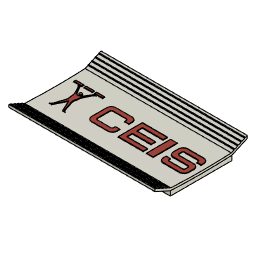
Pen_holder_ceis (Autodesk Fusion 360 design; units mm, degrees)
Autodesk Fusion 360 part; units mm, degrees
sketch "Schizzo3" plane through (0, 0, 0) normal (0, 0, 1) x (1, 0, 0)
  line L0 (0, 0) -> (190, 0)
  line L1 (190, 0) -> (190, 80)
  line L2 (190, 80) -> (0, 80)
  line L3 (0, 80) -> (0, 0)
  dimension "d7" = 80
  dimension "d8" = 190
  constraint horizontal L0
  constraint vertical L1
  constraint horizontal L2
  constraint vertical L3
  constraint coincident L0.start L3.end
  measures "d7" distance of L0.start L2.end
  measures "d8" distance of L1.end L2.end
extrude "Estrusione2" add sketch "Schizzo3" along normal blind 6 makes body 1
sketch "Schizzo4" plane through (190, 0, 0) normal (1, 0, 0) x (0, 1, 0)
  line L0 (0, 0) -> (80, 0)
  line L1 (80, 0) -> (80, 6)
  line L2 (80, 6) -> (0, 6)
  line L3 (0, 6) -> (0, 0)
  line L4 (0, 6) -> (0, 5)
  line L5 (40, 5) -> (40, 9)
  line L6 (-6.5555, 6.3549) -> (30, 25)
  line L7 (30, 25) -> (86.5555, 6.3549)
  arc A0 (-6.5555, 6.3549) -> (86.5555, 6.3549) centre (40, 805.5001) ccw
  constraint coincident L2.end L3.start
  constraint coincident L3 L4.end
  constraint perpendicular L2 L4
  constraint perpendicular L2 L5
  constraint coincident L5.start A0
  constraint coincident L1.end A0
  constraint coincident L2.end A0
extrude "Estrusione3" cut sketch "Schizzo4" against normal through all contours L2 L5 A0 | L2 L6 L7 A0 | L2 L5 A0 bodies 1
sketch "Schizzo5" plane through (190, 0, 0) normal (1, 0, 0) x (0, 1, 0)
  line L0 (80, 0) -> (80, 6)
  line L1 (0, 0) -> (-20, 0)
  line L2 (-20, 0) -> (-20, 15)
  line L3 (80, 0) -> (100, 0)
  line L4 (100, 0) -> (100, 15)
  line L5 (-20, 15) -> (0, 6)
  line L6 (100, 15) -> (80, 6)
  spline S0 degree 5 poles (0, 6) (1.6, 5.9242) (4.8, 5.7791) (9.6, 5.5813) (16, 5.3581) (24, 5.1509) (32, 5.0221) (40, 4.978) (48, 5.0221) (56, 5.1509) (64, 5.3581) (70.4, 5.5813) (75.2, 5.7791) (78.4, 5.9242) (80, 6) knots 0 0 0 0 0 0 0.1 0.2 0.3 0.4 0.5 0.6 0.7 0.8 0.9 1 1 1 1 1 1
  line L7 (-20, 15) -> (-20, 18.2898)
  line L8 (100, 15) -> (100, 18.2898)
  line L9 (-18.7689, 17.7358) -> (0.7109, 8.9698)
  spline S1 degree 3 poles (0.7109, 8.9698) (18.3427, 8.1444) (35.9568, 7.8068) (53.5771, 8.1239) (62.1442, 8.2781) (70.7163, 8.5685) (79.2891, 8.9698) knots 0.007133 0.007133 0.007133 0.007133 0.670389 0.670389 0.670389 0.992867 0.992867 0.992867 0.992867
  line L10 (98.7689, 17.7358) -> (79.2891, 8.9698)
  line L11 (98.7689, 17.7358) -> (100, 18.2898)
  line L12 (-18.7689, 17.7358) -> (-20, 18.2898)
  line L13 (0.7109, 8.9698) -> (-2.9367, 10.6113)
  line L14 (-2.9367, 10.6113) -> (-2.7316, 11.0673)
  line L15 (-2.7316, 11.0673) -> (-3.6435, 11.4776)
  line L16 (-3.6435, 11.4776) -> (-3.8487, 11.0217)
  line L17 (-3.8487, 11.0217) -> (-7.4964, 12.6631)
  line L18 (-7.4964, 12.6631) -> (-7.2912, 13.1191)
  line L19 (-7.2912, 13.1191) -> (-8.2031, 13.5294)
  line L20 (-8.2031, 13.5294) -> (-8.4083, 13.0735)
  line L21 (-8.4083, 13.0735) -> (-12.056, 14.7149)
  line L22 (-12.056, 14.7149) -> (-11.8508, 15.1709)
  line L23 (-11.8508, 15.1709) -> (-12.7627, 15.5813)
  line L24 (-12.7627, 15.5813) -> (-12.9679, 15.1253)
  line L25 (-12.9679, 15.1253) -> (-16.6156, 16.7668)
  line L26 (-16.6156, 16.7668) -> (-16.4104, 17.2227)
  line L27 (-16.4104, 17.2227) -> (-17.3223, 17.6331)
  line L28 (-17.3223, 17.6331) -> (-17.5275, 17.1771)
  line L29 (0, 0) -> (40, 0)
  line L30 (40, 0) -> (40, -6)
  line L31 (82.9368, 10.6113) -> (82.7316, 11.0673)
  line L32 (82.7316, 11.0673) -> (83.6435, 11.4776)
  line L33 (83.6435, 11.4776) -> (83.8487, 11.0217)
  line L34 (87.2912, 13.1191) -> (88.2031, 13.5294)
  line L35 (87.4964, 12.6631) -> (87.2912, 13.1191)
  line L36 (88.2031, 13.5294) -> (88.4083, 13.0735)
  line L37 (92.056, 14.7149) -> (91.8508, 15.1709)
  line L38 (91.8508, 15.1709) -> (92.7627, 15.5813)
  line L39 (92.7627, 15.5813) -> (92.9679, 15.1253)
  line L40 (96.6156, 16.7668) -> (96.4104, 17.2227)
  line L41 (96.4104, 17.2227) -> (97.3223, 17.6331)
  line L42 (97.3223, 17.6331) -> (97.5275, 17.1771)
  point P0 (40, 5)
  dimension "d18" = 20
  dimension "d19" = 15
  dimension "d20" = 20
  dimension "d22" = 15
  dimension "d37" = 3
  dimension "d38" = 4
  dimension "d39" = 0.5
  dimension "d40" = 1
  dimension "d41" = 0.5
  dimension "d42" = 4
  dimension "d43" = 0.5
  dimension "d44" = 1
  dimension "d45" = 0.5
  dimension "d46" = 4
  dimension "d47" = 0.5
  dimension "d48" = 1
  dimension "d49" = 0.5
  dimension "d50" = 4
  dimension "d51" = 0.5
  dimension "d52" = 1
  dimension "d53" = 0.5
  constraint coincident L1.start L29.start
  constraint horizontal L1
  constraint perpendicular L1 L2
  constraint coincident L0.start L3.start
  constraint perpendicular L0 L3
  constraint perpendicular L3 L4
  constraint coincident L0.end L6.end
  constraint parallel L2 L7
  constraint parallel L4 L8
  constraint parallel L10 L11
  constraint parallel L9 L12
  constraint parallel L9 L13
  constraint perpendicular L9 L14
  constraint perpendicular L14 L15
  constraint perpendicular L15 L16
  constraint perpendicular L16 L17
  constraint perpendicular L17 L18
  constraint perpendicular L18 L19
  constraint perpendicular L19 L20
  constraint perpendicular L20 L21
  constraint perpendicular L9 L22
  constraint perpendicular L22 L23
  constraint perpendicular L23 L24
  constraint perpendicular L24 L25
  constraint perpendicular L9 L26
  constraint perpendicular L26 L27
  constraint perpendicular L27 L28
  constraint parallel L1 L29
  constraint perpendicular L29 L30
  constraint symmetric L13.end L30 L31.start
  constraint symmetric L14.end L30 L31.end
  constraint symmetric L15.end L30 L32.end
  constraint symmetric L16.end L30 L33.end
  constraint symmetric L17.end L30 L35.start
  constraint symmetric L18.end L30 L34.start
  constraint symmetric L19.end L30 L34.end
  constraint symmetric L20.end L30 L36.end
  constraint symmetric L21.end L30 L37.start
  constraint symmetric L22.end L30 L37.end
  constraint symmetric L23.end L30 L38.end
  constraint symmetric L24.end L30 L39.end
  constraint symmetric L25.end L30 L40.start
  constraint symmetric L26.end L30 L40.end
  constraint symmetric L27.end L30 L41.end
  constraint symmetric L28.end L30 L42.end
  measures "d18" distance of L1.start L1.end
  measures "d19" distance of L1.end L2.end
  measures "d20" distance of L0.start L3.end
  measures "d22" distance of L3.end L4.end
  measures "d38" distance of L9.end L13.end
  measures "d39" distance of L13.end L14.end
  measures "d40" distance of L14.end L15.end
  measures "d41" distance of L15.end L16.end
  measures "d42" distance of L16.end L17.end
  measures "d43" distance of L17.end L18.end
  measures "d44" distance of L18.end L19.end
  measures "d45" distance of L19.end L20.end
  measures "d46" distance of L20.end L21.end
  measures "d47" distance of L21.end L22.end
  measures "d48" distance of L22.end L23.end
  measures "d49" distance of L23.end L24.end
  measures "d50" distance of L24.end L25.end
  measures "d51" distance of L25.end L26.end
  measures "d52" distance of L26.end L27.end
  measures "d53" distance of L27.end L28.end
extrude "Estrusione5" add sketch "Schizzo5" against normal blind 190 separate body contours L5 L6 S0 L7 L8 L9 S1 L10 L11 L12 L13 L17 L21 L25 | L10 L40 L41 L42 | L9 L26 L27 L28 | L10 L37 L38 L39 | L9 L22 L23 L24 | L10 L34 L35 L36 | L9 L18 L19 L20 | L10 L31 L32 L33 | L9 L14 L15 L16 makes body 2
ref_plane "Piano di lavoro1" through (0, 0, 10) normal (0, 0, 1) x (1, 0, 0)
sketch "Schizzo8" plane through (0, 0, 10) normal (0, 0, 1) x (1, 0, 0)
  arc A0 (63.5, 56) -> (57.5, 50) centre (63.5, 50) ccw
  arc A1 (84.5, 48.2) -> (82.7, 50) centre (82.7, 48.2) ccw
  arc A2 (63.5, 32) -> (65.3, 30.2) centre (65.3, 32) ccw
  arc A3 (84.5, 24.2) -> (90.5, 30.2) centre (84.5, 30.2) ccw
  line L0 (63.5, 24.2) -> (84.5, 24.2)
  line L1 (63.5, 30.2) -> (65.3, 30.2)
  arc A4 (65.3, 50) -> (63.5, 48.2) centre (65.3, 48.2) ccw
  line L2 (57.5, 50) -> (90.5, 50)
  line L3 (57.5, 50) -> (57.5, 30.2)
  line L4 (57.5, 30.2) -> (90.5, 30.2)
  line L5 (84.5, 56) -> (63.5, 56)
  arc A5 (90.5, 50) -> (84.5, 56) centre (84.5, 50) ccw
  arc A6 (82.7, 30.2) -> (84.5, 32) centre (82.7, 32) ccw
  arc A7 (57.5, 30.2) -> (63.5, 24.2) centre (63.5, 30.2) ccw
  line L6 (84.5, 32) -> (82.7, 32)
  line L7 (84.5, 45.8) -> (90.5, 45.8)
  line L8 (63.5, 56) -> (63.5, 24.2)
  line L9 (84.5, 34.4) -> (90.5, 34.4)
  line L10 (103.5, 24.2) -> (103.5, 56)
  line L11 (97.5, 50) -> (130.5006, 50)
  line L12 (97.5, 43.1) -> (127.823, 43.1)
  line L13 (97.5, 40.1) -> (127.823, 40.1)
  line L14 (97.5, 37.1) -> (127.823, 37.1)
  line L15 (97.5, 24.2) -> (97.5, 56)
  line L16 (97.5, 24.2) -> (97.5, 49.1)
  line L17 (97.5, 56) -> (97.5, 40.1)
  line L18 (97.5, 30.2) -> (130.5, 30.2)
  line L19 (97.5, 24.2) -> (130.5, 24.2)
  line L20 (130.5, 24.2) -> (97.5, 24.2)
  line L21 (127.823, 37.1) -> (127.823, 43.1)
  line L22 (97.5, 56) -> (130.5, 56)
  line L23 (134.5, 41.008) -> (134.5, 24.2)
  line L24 (134.5, 39.175) -> (134.5, 55.9829)
  line L25 (143.5, 24.2) -> (143.5, 40.0915)
  line L26 (143.5, 40.0915) -> (143.5, 55.9829)
  arc A8 (177.5, 35.3) -> (175.7, 37.1) centre (175.7, 35.3) ccw
  line L27 (156.5, 37.1) -> (177.5, 37.1)
  line L28 (177.5, 43.1) -> (156.5, 43.1)
  line L29 (150.5, 50) -> (183.5, 50)
  arc A9 (156.5, 55.9397) -> (150.5603, 50) centre (156.5, 50) ccw
  line L30 (177.5, 56) -> (155.5, 56)
  arc A10 (183.5, 49.999) -> (177.5, 56) centre (177.5, 50) ccw
  arc A11 (183.5, 37.0982) -> (177.5, 43.1) centre (177.5, 37.1) ccw
  arc A12 (177.5, 48.2) -> (175.7, 50) centre (175.7, 48.2) ccw
  line L31 (177.5, 46.4) -> (183.5, 46.4)
  arc A13 (156.5, 44.9) -> (158.3, 43.1) centre (158.3, 44.9) ccw
  arc A14 (150.5, 43.1015) -> (156.5, 37.1) centre (156.5, 43.1) ccw
  line L32 (150.5, 30.2) -> (183.5, 30.2)
  line L33 (155.5, 24.2) -> (177.5, 24.2)
  arc A15 (150.5, 30.2) -> (156.5, 24.2) centre (156.5, 30.2) ccw
  arc A16 (156.5, 32) -> (158.3, 30.2) centre (158.3, 32) ccw
  line L34 (150.5, 33.8) -> (156.5, 33.8)
  arc A17 (177.5, 24.2) -> (183.5, 30.201) centre (177.5, 30.2) ccw
  line L35 (134.5, 55.9829) -> (143.5, 55.9829)
  line L36 (134.5, 24.2) -> (143.5, 24.2)
  line L37 (130.5, 56) -> (130.5006, 50)
  line L38 (130.5, 30.2) -> (130.5, 24.2)
  line L39 (84.5, 56) -> (84.5, 45.8)
  line L40 (84.5, 34.4) -> (84.5, 24.2)
  line L41 (90.5, 30.2) -> (90.5, 34.4)
  line L42 (90.5, 45.8) -> (90.5, 50)
  line L43 (150.5, 50) -> (150.5, 43.0985)
  line L44 (150.5, 33.8) -> (150.5, 30.2)
  line L45 (156.5, 56) -> (156.5, 37.1)
  line L46 (156.5, 33.8) -> (156.5, 24.2)
  line L47 (177.5, 24.2) -> (177.5, 43.1)
  line L48 (177.5, 46.4) -> (177.5, 56)
  line L49 (183.5, 30.199) -> (183.5, 37.1018)
  line L50 (183.5, 46.4) -> (183.5, 50.001)
  line L51 (6.5, 60.5) -> (17.5, 60.5)
  line L52 (17.5, 60.5) -> (17.5, 57.5)
  line L53 (17.5, 57.5) -> (6.5, 57.5)
  line L54 (6.5, 57.5) -> (6.5, 60.5)
  circle A18 centre (25.5, 48) radius 2
  line L55 (25.5, 48) -> (25.5, 66.722)
  line L56 (20, 57.5) -> (25.5, 57.5)
  line L57 (25.5, 57.5) -> (25.5, 60.5)
  line L58 (25.5, 60.5) -> (20, 60.5)
  line L59 (20, 60.5) -> (20, 57.5)
  line L60 (3, 16.5) -> (25.5, 16.5)
  line L61 (25.5, 16.5) -> (25.5, 62.5012)
  line L62 (25.5, 62.5012) -> (3, 62.5012)
  line L63 (3, 62.5012) -> (3, 16.5)
  line L64 (13.5, 56.5) -> (16.5, 56.5)
  line L65 (16.5, 56.5) -> (17, 55)
  line L66 (17, 55) -> (22.5, 46)
  line L67 (22.5, 46) -> (25.5, 45)
  line L68 (13.5, 56.5) -> (16, 54.5)
  line L69 (16, 54.5) -> (21, 44.5)
  line L70 (21, 44.5) -> (22.5, 34.5)
  line L71 (22.5, 34.5) -> (17.5, 19.5)
  line L72 (17.5, 19.5) -> (15, 17.5)
  line L73 (15, 17.5) -> (18.5, 17.5)
  line L74 (18.5, 17.5) -> (25.5, 32.5)
  line L75 (25.5, 60.5) -> (31, 60.5)
  line L76 (31, 60.5) -> (31, 57.5)
  line L77 (31, 57.5) -> (25.5, 57.5)
  line L78 (33.5, 60.5) -> (33.5, 57.5)
  line L79 (44.5, 60.5) -> (33.5, 60.5)
  line L80 (44.5, 57.5) -> (44.5, 60.5)
  line L81 (33.5, 57.5) -> (44.5, 57.5)
  line L82 (37.5, 56.5) -> (34.5, 56.5)
  line L83 (34.5, 56.5) -> (34, 55)
  line L84 (34, 55) -> (28.5, 46)
  line L85 (37.5, 56.5) -> (35, 54.5)
  line L86 (35, 54.5) -> (30, 44.5)
  circle A19 centre (25.5, 48) radius 2
  line L87 (28.5, 46) -> (25.5, 45)
  line L88 (30, 44.5) -> (28.5, 34.5)
  line L89 (28.5, 34.5) -> (33.5, 19.5)
  line L90 (32.5, 17.5) -> (25.5, 32.5)
  line L91 (36, 17.5) -> (32.5, 17.5)
  line L92 (33.5, 19.5) -> (36, 17.5)
  line L93 (25.5, 62.5012) -> (48, 62.5012)
  line L94 (48, 62.5012) -> (48, 16.5)
  line L95 (48, 16.5) -> (25.5, 16.5)
  point P0 (143.5, 55.9829)
  point P1 (158.3, 48.2)
  point P2 (177.5, 37.1)
  point P3 (156.5, 48.2)
  point P4 (158.3, 50)
  point P5 (117.5, -48.5)
  point P6 (150.6297, 56)
  constraint horizontal L0
  constraint vertical L41
  constraint horizontal L5
  constraint vertical L3
  constraint perpendicular L0 L8
  constraint perpendicular L5 L39
  constraint perpendicular L2 L41
  constraint perpendicular L4 L41
  constraint coincident A0.centre L8
  constraint coincident A0.centre L2
  constraint coincident A5.centre L2
  constraint coincident A5.centre L39
  constraint coincident L1.start L8
  constraint coincident L1.start L4
  constraint coincident A3.centre L4
  constraint coincident A3.centre L39
  constraint coincident L1.start A7.centre
  constraint perpendicular L1 L8
  constraint tangent A2 L8
  constraint coincident A6.end L39
  constraint perpendicular L6 L39
  constraint coincident A6.centre L6.end
  constraint tangent A1 L2
  constraint coincident A4.end L8
  constraint coincident A4.start L2
  constraint coincident A2.start L8
  constraint coincident A6.start L4
  constraint coincident A1.end L2
  constraint coincident A1.start L39
  constraint coincident L7.end L41
  constraint perpendicular L7 L41
  constraint coincident L9.start L39
  constraint perpendicular L9 L41
  constraint perpendicular L16 L19
  constraint horizontal L20
  constraint coincident L10.start L19
  constraint horizontal L11
  constraint coincident L11.start L15
  constraint coincident L11.start L17
  constraint coincident L18.start L16
  constraint coincident L18.start L15
  constraint coincident L14.start L15
  constraint coincident L13.start L15
  constraint parallel L12 L13
  constraint coincident P0 L26.end
  constraint horizontal L33
  constraint vertical L49
  constraint horizontal L30
  constraint vertical L43
  constraint coincident L29.end L49
  constraint perpendicular L29 L49
  constraint coincident L32.end L49
  constraint perpendicular L32 L49
  constraint coincident P6 L30
  constraint coincident L45.start L30
  constraint perpendicular L32 L45
  constraint perpendicular L30 L47
  constraint coincident A9.centre L45
  constraint coincident A9.centre L29
  constraint coincident A17.centre L47
  constraint coincident A17.centre L32
  constraint coincident A10.centre L47
  constraint coincident A10.centre L29
  constraint coincident L34.start L43
  constraint coincident L34.end L45
  constraint perpendicular L34 L45
  constraint coincident L31.start L47
  constraint coincident L31.end L49
  constraint coincident A9.start L45
  constraint coincident A9.end L29
  constraint coincident A17.end L49
  constraint coincident A10.start L49
  constraint tangent L29 A12
  constraint coincident P3 L45
  constraint coincident P4 L29
  constraint coincident A12.end L29
  constraint coincident A12.start L47
  constraint coincident A16.end L32
  constraint coincident A16.start L45
  constraint perpendicular L28 L47
  constraint coincident L28.end L45
  constraint coincident P2 L47
  constraint perpendicular L27 L47
  constraint tangent A8 L27
  constraint coincident L28.end A14.centre
  constraint coincident P2 L27.end
  constraint coincident A14.start L43
  constraint coincident A11.start L49
  constraint coincident A8.end L27
  constraint coincident A8.start L47
  constraint coincident A13.end L28
  constraint coincident A13.start L45
  constraint perpendicular L26 L35
  constraint perpendicular L25 L36
  constraint perpendicular L20 L38
  constraint coincident L21 L13.end
  constraint collinear L39 L40
  constraint collinear L41 L42
  constraint coincident A17 L49.start
  constraint coincident A10 L50.end
  constraint coincident A14 L43.end
  constraint collinear L43 L44
  constraint collinear L45 L46
  constraint collinear L47 L48
  constraint coincident A11 L49.end
  constraint collinear L49 L50
  constraint horizontal L51
  constraint vertical L52
  constraint horizontal L53
  constraint vertical L54
  constraint coincident A18.centre L55.start
  constraint horizontal L56
  constraint vertical L57
  constraint horizontal L58
  constraint vertical L59
  constraint coincident L55 L57.end
  constraint horizontal L60
  constraint vertical L61
  constraint horizontal L62
  constraint vertical L63
  constraint coincident L55 L61.end
  constraint parallel L53 L64
  constraint coincident L61 L67.end
  constraint horizontal L73
  constraint coincident L61 L74.end
  constraint symmetric L51.start L61 L79.start
  constraint symmetric L51.end L61 L78.start
  constraint symmetric L52.end L61 L78.end
  constraint symmetric L53.end L61 L80.start
  constraint symmetric A18 L61 A19
  constraint symmetric L56.start L61 L76.end
  constraint symmetric L56.end L61 L57.start
  constraint symmetric L57.end L61 L58.start
  constraint symmetric L58.end L61 L75.end
  constraint symmetric L61 L64.start L82.start
  constraint symmetric L61 L64.end L82.end
  constraint symmetric L61 L65.end L83.end
  constraint symmetric L61 L66.end L84.end
  constraint symmetric L61 L67.end L87.end
  constraint symmetric L61 L68.end L85.end
  constraint symmetric L61 L69.end L86.end
  constraint symmetric L61 L70.end L88.end
  constraint symmetric L61 L71.end L89.end
  constraint symmetric L61 L72.end L91.start
  constraint symmetric L61 L73.end L90.start
  constraint symmetric L61 L74.end L90.end
  constraint symmetric L55 L60.start L94.end
  constraint symmetric L55 L60.end L61.start
  constraint symmetric L55 L61.end L62.start
  constraint symmetric L55 L62.end L93.end
extrude "Estrusione6" cut sketch "Schizzo8" against normal blind 4 contours A0 L2 L8 | L2 L5 L8 L39 | L2 L3 L4 L8 | L2 A5 L39 | A4 L2 L8 | L4 A7 L8 | L2 L7 L39 L42 | A1 L2 L39 | A2 L1 L4 L8 | L0 L1 L4 L8 L40 | A3 L4 L40 | L4 A6 L40 | L4 L9 L40 L41 | L10 L15 L16 L18 L19 L20 | L10 L18 L19 L20 L38 | L10 L14 L15 L16 L18 | L10 L13 L14 L15 L16 | L10 L13 L14 L21 | L10 L12 L13 L15 L16 L17 | L10 L12 L13 L21 | L10 L11 L12 L15 L16 L17 | L10 L11 L15 L17 L22 | L10 L11 L22 L37 | L23 L24 L25 L26 L35 L36 | A8 L27 L47 | A11 L32 L47 L49 | L27 L28 L45 L47 | L32 L33 L46 L47 | L32 A17 L47 | L29 A14 L43 L45 | L32 A16 L46 | L28 A13 L45 | L32 A15 L46 | L32 L34 L44 L46 | L29 L30 L45 L48 | L29 A9 L45 | L29 A12 L48 | L29 A10 L48 | L29 L31 L48 L50 | L51 L52 L53 L54 | A18 L55 L61 A19 | A18 L55 L61 A19 | L55 L56 L57 L58 L59 L61 | L55 L57 L61 L75 L76 L77 | L61 L82 L83 L84 L85 L86 L87 L88 L89 L90 L91 L92 | L61 L64 L65 L66 L67 L68 L69 L70 L71 L72 L73 L74 | L78 L79 L80 L81 bodies 2
sketch "Schizzo10" plane through (0, 0, 0) normal (0, 0, 1) x (1, 0, 0)
  arc A0 (383.5, 49.999) -> (377.5, 56) centre (377.5, 50) ccw
  line L0 (327.823, 37.1) -> (327.823, 43.1)
  line L1 (383.5, 46.4) -> (383.5, 50.001)
  line L2 (377.5, 32) -> (377.5, 35.3)
  line L3 (221, 44.5) -> (222.5, 34.5)
  line L4 (297.5, 24.2) -> (297.5, 49.1)
  line L5 (257.5, 50) -> (257.5, 30.2)
  line L6 (377.5, 46.4) -> (377.5, 48.2)
  line L7 (297.5, 24.2) -> (330.5, 24.2)
  line L8 (383.5, 30.199) -> (383.5, 37.1018)
  line L9 (303.5, 30.2) -> (330.5, 30.2)
  arc A1 (350.5, 30.2) -> (356.5, 24.2) centre (356.5, 30.2) ccw
  line L10 (334.5, 24.2) -> (343.5, 24.2)
  line L11 (343.5, 24.2) -> (343.5, 40.0915)
  line L12 (350.5, 33.8) -> (356.5, 33.8)
  line L13 (356.5, 37.1) -> (375.7, 37.1)
  line L14 (303.5, 37.1) -> (327.823, 37.1)
  line L15 (330.5, 30.2) -> (330.5, 24.2)
  line L16 (356.5, 24.2) -> (377.5, 24.2)
  line L17 (334.5, 41.008) -> (334.5, 24.2)
  arc A2 (284.5, 48.2) -> (282.7, 50) centre (282.7, 48.2) ccw
  arc A3 (263.5, 56) -> (257.5, 50) centre (263.5, 50) ccw
  arc A4 (377.5, 48.2) -> (375.7, 50) centre (375.7, 48.2) ccw
  line L18 (330.5, 56) -> (330.5006, 50)
  line L19 (350.5, 33.8) -> (350.5, 30.2)
  line L20 (284.5, 45.8) -> (290.5, 45.8)
  arc A5 (265.3, 50) -> (263.5, 48.2) centre (265.3, 48.2) ccw
  line L21 (290.5, 45.8) -> (290.5, 50)
  line L22 (218.5, 17.5) -> (225.5, 32.5)
  arc A6 (377.5, 24.2) -> (383.5, 30.201) centre (377.5, 30.2) ccw
  line L23 (217.5, 60.5) -> (217.5, 57.5)
  arc A7 (263.5, 32) -> (265.3, 30.2) centre (265.3, 32) ccw
  line L24 (233.5, 60.5) -> (233.5, 57.5)
  line L25 (244.5, 57.5) -> (244.5, 60.5)
  line L26 (233.5, 57.5) -> (244.5, 57.5)
  arc A8 (356.5, 44.9) -> (358.3, 43.1) centre (358.3, 44.9) ccw
  line L27 (303.5, 50) -> (330.5006, 50)
  arc A9 (290.5, 50) -> (284.5, 56) centre (284.5, 50) ccw
  arc A10 (377.5, 35.3) -> (375.7, 37.1) centre (375.7, 35.3) ccw
  line L28 (290.5, 30.2) -> (290.5, 34.4)
  line L29 (233.5, 19.5) -> (236, 17.5)
  line L30 (297.5, 24.2) -> (297.5, 56)
  circle A11 centre (225.5, 48) radius 2
  arc A12 (282.7, 30.2) -> (284.5, 32) centre (282.7, 32) ccw
  line L31 (330.5, 24.2) -> (297.5, 24.2)
  line L32 (284.5, 48.2) -> (284.5, 45.8)
  arc A13 (356.5, 32) -> (358.3, 30.2) centre (358.3, 32) ccw
  line L33 (350.5, 50) -> (350.5, 43.0985)
  line L34 (284.5, 56) -> (263.5, 56)
  line L35 (217, 55) -> (222.5, 46)
  line L36 (217.5, 19.5) -> (215, 17.5)
  line L37 (206.5, 57.5) -> (206.5, 60.5)
  line L38 (228.5, 46) -> (225.5, 45)
  line L39 (265.3, 30.2) -> (282.7, 30.2)
  line L40 (220, 60.5) -> (220, 57.5)
  line L41 (237.5, 56.5) -> (235, 54.5)
  line L42 (206.5, 60.5) -> (217.5, 60.5)
  line L43 (232.5, 17.5) -> (225.5, 32.5)
  line L44 (234, 55) -> (228.5, 46)
  line L45 (231, 60.5) -> (231, 57.5)
  line L46 (217.5, 57.5) -> (206.5, 57.5)
  line L47 (216.5, 56.5) -> (217, 55)
  line L48 (222.5, 34.5) -> (217.5, 19.5)
  line L49 (234.5, 56.5) -> (234, 55)
  line L50 (263.5, 24.2) -> (284.5, 24.2)
  line L51 (225.5, 60.5) -> (220, 60.5)
  line L52 (213.5, 56.5) -> (216.5, 56.5)
  arc A14 (257.5, 30.2) -> (263.5, 24.2) centre (263.5, 30.2) ccw
  line L53 (216, 54.5) -> (221, 44.5)
  circle A15 centre (225.5, 48) radius 2
  line L54 (225.5, 60.5) -> (231, 60.5)
  line L55 (237.5, 56.5) -> (234.5, 56.5)
  line L56 (222.5, 46) -> (225.5, 45)
  line L57 (235, 54.5) -> (230, 44.5)
  line L58 (236, 17.5) -> (232.5, 17.5)
  line L59 (213.5, 56.5) -> (216, 54.5)
  line L60 (231, 57.5) -> (225.5, 57.5)
  line L61 (220, 57.5) -> (225.5, 57.5)
  line L62 (284.5, 34.4) -> (290.5, 34.4)
  line L63 (244.5, 60.5) -> (233.5, 60.5)
  arc A16 (284.5, 24.2) -> (290.5, 30.2) centre (284.5, 30.2) ccw
  line L64 (215, 17.5) -> (218.5, 17.5)
  line L65 (228.5, 34.5) -> (233.5, 19.5)
  line L66 (303.5, 43.1) -> (327.823, 43.1)
  line L67 (377.5, 56) -> (356.5, 56)
  arc A17 (383.5, 37.0982) -> (377.5, 43.1) centre (377.5, 37.1) ccw
  line L68 (265.3, 50) -> (282.7, 50)
  line L69 (377.5, 43.1) -> (358.3, 43.1)
  line L70 (343.5, 40.0915) -> (343.5, 55.9829)
  line L71 (297.5, 56) -> (297.5, 40.1)
  line L72 (377.5, 46.4) -> (383.5, 46.4)
  arc A18 (350.5, 43.1015) -> (356.5, 37.1) centre (356.5, 43.1) ccw
  line L73 (334.5, 55.9829) -> (343.5, 55.9829)
  line L74 (297.5, 56) -> (330.5, 56)
  line L75 (334.5, 39.175) -> (334.5, 55.9829)
  line L76 (230, 44.5) -> (228.5, 34.5)
  line L77 (284.5, 34.4) -> (284.5, 32)
  line L78 (263.5, 48.2) -> (263.5, 32)
  line L79 (303.5, 30.2) -> (303.5, 37.1)
  line L80 (303.5, 43.1) -> (303.5, 50)
  line L81 (356.5, 56) -> (356.5, 55.9397)
  line L82 (358.3, 50) -> (375.7, 50)
  line L83 (356.5, 48.2005) -> (356.5, 44.9)
  line L84 (356.5, 33.8) -> (356.5, 32)
  line L85 (358.3, 30.2) -> (375.7, 30.2)
  arc A19 (375.7, 30.2) -> (377.5, 32) centre (375.7, 32) ccw
  arc A20 (358.3, 50) -> (356.5, 48.2) centre (358.3, 48.2) ccw
  line L86 (222.3674, 45.8334) -> (225.5, 44.7892)
  line L87 (228.6326, 45.8334) -> (225.5, 44.7892)
  line L88 (234.1825, 54.9151) -> (228.6326, 45.8334)
  line L89 (234.6442, 56.3) -> (234.1825, 54.9151)
  line L90 (236.9298, 56.3) -> (234.6442, 56.3)
  line L91 (236.9298, 56.3) -> (234.8408, 54.6287)
  line L92 (234.8408, 54.6287) -> (229.8069, 44.5611)
  line L93 (229.8069, 44.5611) -> (228.2951, 34.4822)
  line L94 (228.2951, 34.4822) -> (233.3289, 19.3807)
  line L95 (233.3289, 19.3807) -> (235.4298, 17.7)
  line L96 (235.4298, 17.7) -> (232.6274, 17.7)
  line L97 (232.6274, 17.7) -> (225.5, 32.9729)
  line L98 (218.3726, 17.7) -> (225.5, 32.9729)
  line L99 (215.5702, 17.7) -> (218.3726, 17.7)
  line L100 (217.6711, 19.3807) -> (215.5702, 17.7)
  line L101 (222.7049, 34.4822) -> (217.6711, 19.3807)
  line L102 (221.1931, 44.5611) -> (222.7049, 34.4822)
  line L103 (216.1592, 54.6287) -> (221.1931, 44.5611)
  line L104 (214.0702, 56.3) -> (216.1592, 54.6287)
  line L105 (214.0702, 56.3) -> (216.3558, 56.3)
  line L106 (216.3558, 56.3) -> (216.8175, 54.9151)
  line L107 (216.8175, 54.9151) -> (222.3674, 45.8334)
  circle A21 centre (225.5, 48) radius 1.8
  line L108 (220.2, 57.7) -> (225.5, 57.7)
  line L109 (230.8, 57.7) -> (225.5, 57.7)
  line L110 (230.8, 60.3) -> (230.8, 57.7)
  line L111 (225.5, 60.3) -> (230.8, 60.3)
  line L112 (225.5, 60.3) -> (220.2, 60.3)
  line L113 (220.2, 60.3) -> (220.2, 57.7)
  line L114 (217.3, 57.7) -> (206.7, 57.7)
  line L115 (206.7, 57.7) -> (206.7, 60.3)
  line L116 (206.7, 60.3) -> (217.3, 60.3)
  line L117 (217.3, 60.3) -> (217.3, 57.7)
  line L118 (233.7, 57.7) -> (244.3, 57.7)
  line L119 (244.3, 57.7) -> (244.3, 60.3)
  line L120 (244.3, 60.3) -> (233.7, 60.3)
  line L121 (233.7, 60.3) -> (233.7, 57.7)
  line L122 (383.3, 46.6) -> (383.3, 50.001)
  line L123 (377.7, 46.6) -> (383.3, 46.6)
  line L124 (377.7, 46.6) -> (377.7, 48.2)
  arc A22 (377.7, 48.2) -> (375.7, 50.2) centre (375.7, 48.2) ccw
  line L125 (358.3, 50.2) -> (375.7, 50.2)
  arc A23 (358.3, 50.2) -> (356.3, 48.2) centre (358.3, 48.2) ccw
  arc A24 (383.3, 49.999) -> (377.5, 55.8) centre (377.5, 50) ccw
  line L126 (377.5, 55.8) -> (356.5, 55.8)
  arc A25 (362.5, 50) -> (362.4967, 50.2) centre (356.5, 50) ccw
  arc A26 (356.5, 56) -> (350.5, 50) centre (356.5, 50) ccw
  arc A27 (356.5, 55.8) -> (350.7, 50) centre (356.5, 50) ccw
  line L127 (350.7, 50) -> (350.7, 43.0985)
  arc A28 (350.7, 43.1015) -> (356.5, 37.3) centre (356.5, 43.1) ccw
  line L128 (356.5, 37.3) -> (375.7, 37.3)
  arc A29 (377.7, 35.3) -> (375.7, 37.3) centre (375.7, 35.3) ccw
  line L129 (377.7, 32) -> (377.7, 35.3)
  arc A30 (375.7, 30) -> (377.7, 32) centre (375.7, 32) ccw
  line L130 (358.3, 30) -> (375.7, 30)
  arc A31 (356.3, 32) -> (358.3, 30) centre (358.3, 32) ccw
  line L131 (356.3, 33.6) -> (356.3, 32)
  line L132 (350.7, 33.6) -> (356.3, 33.6)
  line L133 (350.7, 33.6) -> (350.7, 30.2)
  arc A32 (350.7, 30.2) -> (356.5, 24.4) centre (356.5, 30.2) ccw
  line L134 (356.5, 24.4) -> (377.5, 24.4)
  arc A33 (377.5, 24.4) -> (383.3, 30.201) centre (377.5, 30.2) ccw
  arc A34 (383.3, 37.0982) -> (377.5, 42.9) centre (377.5, 37.1) ccw
  line L135 (377.5, 42.9) -> (358.3, 42.9)
  arc A35 (356.3, 44.9) -> (358.3, 42.9) centre (358.3, 44.9) ccw
  line L136 (356.3, 48.2005) -> (356.3, 44.9)
  line L137 (383.3, 30.199) -> (383.3, 37.1018)
  line L138 (334.7, 41.008) -> (334.7, 39.175)
  line L139 (334.7, 39.175) -> (334.7, 24.4)
  line L140 (334.7, 24.4) -> (343.3, 24.4)
  line L141 (343.3, 24.4) -> (343.3, 40.0915)
  line L142 (343.3, 40.0915) -> (343.3, 55.7829)
  line L143 (334.7, 55.7829) -> (343.3, 55.7829)
  line L144 (334.7, 41.008) -> (334.7, 55.7829)
  line L145 (297.7, 49.1) -> (297.7, 40.1)
  line L146 (297.7, 55.8) -> (297.7, 49.1)
  line L147 (297.7, 55.8) -> (330.3, 55.8)
  line L148 (330.3, 55.8) -> (330.3006, 50.2)
  line L149 (303.3, 50.2) -> (330.3006, 50.2)
  line L150 (303.3, 42.9) -> (303.3, 50.2)
  line L151 (303.3, 42.9) -> (327.623, 42.9)
  line L152 (327.623, 37.3) -> (327.623, 42.9)
  line L153 (303.3, 37.3) -> (327.623, 37.3)
  line L154 (303.3, 30) -> (303.3, 37.3)
  line L155 (303.3, 30) -> (330.3, 30)
  line L156 (330.3, 30) -> (330.3, 24.4)
  line L157 (297.7, 24.4) -> (330.3, 24.4)
  line L158 (297.7, 24.4) -> (297.7, 40.1)
  line L159 (257.7, 50) -> (257.7, 30.2)
  arc A36 (257.7, 30.2) -> (263.5, 24.4) centre (263.5, 30.2) ccw
  line L160 (263.5, 24.4) -> (284.5, 24.4)
  arc A37 (284.5, 24.4) -> (290.3, 30.2) centre (284.5, 30.2) ccw
  line L161 (290.3, 30.2) -> (290.3, 34.2)
  line L162 (284.7, 34.2) -> (290.3, 34.2)
  line L163 (284.7, 34.2) -> (284.7, 32)
  arc A38 (282.7, 30) -> (284.7, 32) centre (282.7, 32) ccw
  line L164 (265.3, 30) -> (282.7, 30)
  arc A39 (263.3, 32) -> (265.3, 30) centre (265.3, 32) ccw
  line L165 (263.3, 48.2) -> (263.3, 32)
  arc A40 (265.3, 50.2) -> (263.3, 48.2) centre (265.3, 48.2) ccw
  line L166 (265.3, 50.2) -> (282.7, 50.2)
  arc A41 (284.7, 48.2) -> (282.7, 50.2) centre (282.7, 48.2) ccw
  line L167 (284.7, 48.2) -> (284.7, 46)
  line L168 (284.7, 46) -> (290.3, 46)
  line L169 (290.3, 46) -> (290.3, 50)
  arc A42 (290.3, 50) -> (284.5, 55.8) centre (284.5, 50) ccw
  line L170 (284.5, 55.8) -> (263.5, 55.8)
  arc A43 (263.5, 55.8) -> (257.7, 50) centre (263.5, 50) ccw
  point P0 (350.6297, 56)
  point P1 (343.5, 55.9829)
  point P2 (358.3, 48.2)
  point P3 (377.5, 37.1)
  dimension "d85" = 0.2
  dimension "d86" = -0.2
  dimension "d87" = -0.2
  dimension "d88" = 0.2
  dimension "d89" = -0.2
  dimension "d90" = -0.2
  dimension "d91" = -0.2
  dimension "d92" = -0.2
  dimension "d93" = -0.2
  dimension "d94" = -0.2
  dimension "d95" = -0.2
  dimension "d96" = 0.2
  dimension "d97" = 0.2
  dimension "d98" = -0.2
  constraint horizontal L50
  constraint vertical L28
  constraint horizontal L34
  constraint vertical L5
  constraint perpendicular L50 L78
  constraint perpendicular L32 L34
  constraint perpendicular L28 L68
  constraint perpendicular L28 L39
  constraint coincident A14.centre L78
  constraint coincident A16.centre L32
  constraint tangent A7 L78
  constraint coincident A12.end L32
  constraint tangent A2 L68
  constraint coincident L20.end L28
  constraint perpendicular L20 L28
  constraint coincident L62.start L32
  constraint perpendicular L28 L62
  constraint perpendicular L4 L7
  constraint horizontal L31
  constraint horizontal L27
  constraint coincident P1 L70.end
  constraint horizontal L16
  constraint vertical L8
  constraint horizontal L67
  constraint vertical L33
  constraint coincident P0 L67
  constraint perpendicular L2 L67
  constraint coincident A0.centre L2
  constraint coincident L12.start L33
  constraint coincident L12.end L81
  constraint perpendicular L12 L81
  constraint coincident L6.start L2
  constraint coincident L1.start L8
  constraint coincident A6.end L8
  constraint coincident A0.start L8
  constraint coincident A20.end L81
  constraint coincident L6.end L2
  constraint coincident A13.start L81
  constraint perpendicular L2 L69
  constraint perpendicular L2 L13
  constraint tangent L13 A10
  constraint coincident A18.start L33
  constraint coincident A17.start L8
  constraint coincident A8.start L81
  constraint perpendicular L70 L73
  constraint perpendicular L10 L11
  constraint perpendicular L15 L31
  constraint collinear L32 L77
  constraint collinear L21 L28
  constraint coincident L8.start A6
  constraint coincident L1.end A0
  constraint coincident L33.end A18
  constraint collinear L19 L33
  constraint collinear L81 L84
  constraint collinear L2 L6
  constraint coincident L8.end A17
  constraint collinear L1 L8
  constraint horizontal L42
  constraint vertical L23
  constraint horizontal L46
  constraint vertical L37
  constraint horizontal L61
  constraint horizontal L51
  constraint vertical L40
  constraint parallel L46 L52
  constraint horizontal L64
  constraint collinear L79 L80
  constraint collinear L81 L83
  constraint tangent L85 A19
  constraint coincident P2 A20.centre
  constraint tangent L82 A20
  constraint coincident L83.start A20
  constraint coincident L125 A25.end
  constraint concentric A25 A26
  constraint coincident L82 A25.start
extrude "Estrusione9" add sketch "Schizzo10" along normal blind 3 separate body contours L86 L87 L88 L89 L90 L91 L92 L93 L94 L95 L96 L97 L98 L99 L100 L101 L102 L103 L104 L105 L106 L107 | A21 | L108 L109 L110 L111 L112 L113 | L114 L115 L116 L117 | L118 L119 L120 L121 | L122 L123 L124 A22 L125 A23 A24 L126 A27 L127 A28 L128 A29 L129 A30 L130 A31 L131 L132 L133 A32 L134 A33 A34 L135 A35 L136 L137 | L138 L139 L140 L141 L142 L143 L144 | L145 L146 L147 L148 L149 L150 L151 L152 L153 L154 L155 L156 L157 L158 | L159 A36 L160 A37 L161 L162 L163 A38 L164 A39 L165 A40 L166 A41 L167 L168 L169 A42 L170 A43 makes body 3 at (299.5667, 39.1667, 0) makes body 4 at (240.7667, 60.3, 1) makes body 5 at (227.2667, 60.3, 1) makes body 6 at (276.9, 53.9333, 0) makes body 7 at (340.4333, 34.861, 0) makes body 8 at (225.5, 37.9179, 0) makes body 9 at (213.7667, 57.7, 1) makes body 10 at (225.5449, 49.7994, 2) makes body 11 at (369.9, 53.9333, 3)
move_body "Allinea7" bodies 6 to x (1, 0, 0) y (0, 1, 0) z (0, 0, 1) at (-200, -0.2, 5.5866)
move_body "Allinea8" bodies 3 to x (1, 0, 0) y (0, 1, 0) z (0, 0, 1) at (-200, 0.2, 5.5856)
move_body "Allinea9" bodies 7 to x (1, 0, 0) y (0, 1, 0) z (0, 0, 1) at (-200, -0.2, 5.5866)
move_body "Allinea10" bodies 11 to x (1, 0, 0) y (0, 1, 0) z (0, 0, 1) at (-200, 0.2, 5.5856)
move_body "Allinea11" bodies 8 to x (1, 0, 0) y (0, 1, 0) z (0, 0, 1) at (-200.2214, -0.2, 5.6683)
move_body "Allinea12" bodies 5 to x (1, 0, 0) y (0, 1, 0) z (0, 0, 1) at (-213.5, 0.2, 5.6388)
move_body "Allinea13" bodies 9 to x (1, 0, 0) y (0, 1, 0) z (0, 0, 1) at (-186.5, 0.2, 5.6388)
move_body "Allinea14" bodies 4 to x (1, 0, 0) y (0, 1, 0) z (0, 0, 1) at (-200, 0.2, 5.6388)
move_body "Allinea15" bodies 10 to x (1, 0, 0) y (0, -1, 0) z (0, 0, -1) at (-200, 96, 9)
